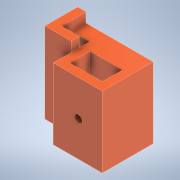
# Autodesk Inventor part: Base Idler Izq
Saved by Autodesk Inventor 2021 (Build 250183000, 183)
## iProperties
Created: 2023-01-27
Part Number: Base Idler Izq
Material: Resina fenólica
Document SubType Name: Modeling
Designer: Diego.labarca
Density: 1.38 g/cm^3
Appearance: Suave - Naranja claro
Author: Diego.labarca
Autodesk Inventor part; units mm, degrees
ref_plane "YZ Plane" through (0, 0, 0) normal (1, 0, 0) x (0, 1, 0)
ref_plane "XZ Plane" through (0, 0, 0) normal (0, 1, 0) x (-1, 0, 0)
ref_plane "XY Plane" through (0, 0, 0) normal (0, 0, 1) x (1, 0, 0)
sketch "Boceto15" plane through (0, 0, 0) normal (1, 0, 0) x (0, 1, 0)
  line L0 (24.65, 10) -> (-24.65, 10)
  line L1 (-24.65, 10) -> (-24.65, -10)
  line L2 (-24.65, -10) -> (24.65, -10)
  line L3 (24.65, -10) -> (24.65, 10)
  line L4 (0, -2.1261) -> (0, 0)
  line L5 (0, 0) -> (1.5481, 0)
  dimension "d52" = 49.3
  dimension "d53" = 20
  constraints: 12 end point, 2 parallel, 2 perpendicular, 1 horizontal, 1 vertical, 2 other
  measures "d52" distance of L2.end L1.end
  measures "d53" distance of L1.end L0.end
extrude "Extrusión12" add sketch "Boceto15" along normal blind 5
sketch "Boceto16" plane through (5, 0, 0) normal (1, 0, 0) x (0, 0, -1)
  circle A0 centre (3.5, -14.65) radius 1.5
  line L0 (10, -24.65) -> (10, 24.65) projected
  line L1 (-10, -24.65) -> (10, -24.65) projected
  circle A1 centre (3.5, 7.35) radius 1.5
  point P0 (0, 0)
  dimension "d56" = 6.5
  dimension "d57" = 10
  dimension "d58" = 3
  dimension "d59" = 3
  dimension "d60" = 32
  dimension "d61" = 6.5
  constraints: 2 centre point
  measures "d56" distance from line of A0.centre L0
  measures "d57" distance from line of L1 A0.centre
  measures "d58" diameter of A0
  measures "d59" diameter of A1
  measures "d60" distance from line of L1 A1.centre
  measures "d61" distance from line of A1.centre L0
extrude "Extrusión13" cut sketch "Boceto16" against normal through all
sketch "Boceto17" plane through (0, -24.65, -10) normal (0, -1, 0) x (1, 0, 0)
  line L0 (5, 20) -> (5, 0) projected
  line L1 (5, 20) -> (16, 20)
  line L2 (16, 20) -> (16, 15)
  line L3 (16, 15) -> (5, 15)
  line L4 (5, 15) -> (5, 20)
  line L5 (16, 15) -> (21, 15)
  line L6 (21, 15) -> (21, 31)
  line L7 (21, 31) -> (16, 31)
  line L8 (16, 31) -> (16, 15)
  line L9 (21, 31) -> (41, 31)
  line L10 (41, 31) -> (41, 26)
  line L11 (41, 26) -> (21, 26)
  line L12 (21, 26) -> (21, 31)
  point P0 (0, 10)
  dimension "d64" = 11
  dimension "d65" = 5
  dimension "d66" = 5
  dimension "d67" = 16
  dimension "d91" = 20
  dimension "d92" = 5
  constraints: 24 end point, 6 parallel, 3 horizontal, 3 perpendicular
  measures "d64" distance of L2.end L3.end
  measures "d65" distance of L1.end L2.end
  measures "d66" distance of L7.end L6.end
  measures "d67" distance of L6.end L5.end
  measures "d91" distance of L10.end L11.end
  measures "d92" distance of L9.end L10.end
extrude "Extrusión14" add sketch "Boceto17" against normal up to surface (49.3 mm away)
sketch "Boceto18" plane through (0, -24.65, 10) normal (0, 0, 1) x (1, 0, 0)
  circle A0 centre (10, 24.3) radius 3.134
  line L0 (0, 0) -> (16, 0) projected
  line L1 (0, 49.3) -> (0, 0) projected
  point P0 (0, 24.65)
  dimension "d70" = 24.3
  dimension "d71" = 10
  constraints: 1 centre point
  measures "d70" distance from line of A0.centre L0
  measures "d71" distance from line of L1 A0.centre
extrude "Extrusión15" cut sketch "Boceto18" against normal up to surface (5 mm away)
sketch "Boceto19" plane through (5, 0, 0) normal (1, 0, 0) x (0, 0, -1)
  line L0 (10, -24.65) -> (10, 24.65) projected
  line L1 (10, -22) -> (7, -22)
  line L2 (7, -22) -> (7, -16)
  line L3 (7, -16) -> (10, -16)
  line L4 (10, -16) -> (10, -22)
  line L5 (10, 9) -> (7, 9)
  line L6 (7, 9) -> (7, 15)
  line L7 (7, 15) -> (10, 15)
  line L8 (10, 15) -> (10, 9)
  line L9 (7, 12) -> (8.4797, 12)
  line L10 (7, -19) -> (9.1788, -19)
  line L11 (-5, -24.65) -> (10, -24.65) projected
  point P0 (0, 0)
  dimension "d74" = 5.65
  dimension "d75" = 6
  dimension "d76" = 6
  dimension "d77" = 31
  dimension "d78" = 3
  constraints: 20 end point, 4 horizontal, 4 parallel, 3 point on line, 2 midpoint, 2 perpendicular
  measures "d74" distance between parallel lines of L11 L10
  measures "d75" distance of L1.end L2.end
  measures "d76" distance of L5.end L6.end
  measures "d77" distance between parallel lines of L10 L9
  measures "d78" distance of L2.end L3.end
extrude "Extrusión16" cut sketch "Boceto19" against normal through all
sketch "Boceto20" plane through (21, -24.65, 5) normal (0, 0, -1) x (-1, 0, 0)
  line L0 (16, 49.3) -> (16, 0) projected
  line L1 (5, 0) -> (5, 49.3) projected
  line L2 (2, 0) -> (2, 49.3)
  line L3 (16, 8.65) -> (16, 33.65) projected
  line L4 (2, 28.65) -> (16, 28.65)
  line L5 (16, 28.65) -> (16, 13.65)
  line L6 (16, 13.65) -> (0, 13.65)
  line L7 (2, 13.65) -> (2, 28.65)
  line L8 (21, 33.65) -> (16, 33.65) projected
  point P0 (2, 13.65)
  dimension "d85" = 5
  dimension "d86" = 15
  dimension "d94" = 14
  constraints: 10 end point, 2 parallel, 2 point on line, 1 horizontal, 1 perpendicular
  measures "d85" distance between parallel lines of L4 L8
  measures "d86" distance between parallel lines of L4 L6
  measures "d94" distance between parallel lines of L0 L7
extrude "Extrusión17" add sketch "Boceto20" along normal up to surface (15 mm away)
sketch "Boceto21" plane through (0, -16, -10) normal (0, 0, -1) x (-1, 0, 0)
  circle A0 centre (-10, 15.65) radius 3.134 projected
  circle A1 centre (-14, 15.65) radius 2
  line L0 (-14, 15.65) -> (-14.5246, 15.65)
  line L1 (-10, 15.65) -> (-9.1195, 15.65)
  line L2 (-21, -8.65) -> (-21, 40.65) projected
  point P0 (0, 16)
  dimension "d87" = 4
  dimension "d106" = 7
  constraints: 4 end point, 2 horizontal, 1 centre point, 1 collinear
  measures "d87" diameter of A1
  measures "d106" distance from line of L2 L0.start
extrude "Extrusión18" cut sketch "Boceto21" against normal blind 7 contours A1 A0 | A0 A1 picked at (-12.7449, 15.65) picked at (-14.0736, 15.5709)
sketch "Boceto22" plane through (0, -24.65, -10) normal (0, -1, 0) x (1, 0, 0)
  line L0 (21, 15) -> (21, 26) projected
  line L1 (21, 13.5) -> (41, 13.5)
  line L2 (41, 13.5) -> (41, 8.5)
  line L3 (41, 8.5) -> (21, 8.5)
  line L4 (21, 8.5) -> (21, 13.5)
  line L5 (21, 26) -> (41, 26) projected
  line L6 (16, 31) -> (16, 20) projected
  line L7 (21, 8.5) -> (16, 8.5)
  line L8 (16, 8.5) -> (16, 20)
  line L9 (16, 20) -> (21, 20)
  line L10 (21, 20) -> (21, 8.5)
  point P0 (0, 10)
  dimension "d95" = 5
  dimension "d96" = 12.5
  constraints: 16 end point, 4 parallel, 2 horizontal, 2 perpendicular, 1 point on line
  measures "d95" distance of L1.end L2.end
  measures "d96" distance between parallel lines of L5 L1
extrude "Extrusión19" add sketch "Boceto22" against normal up to surface (49.3 mm away)
sketch "Boceto24" plane through (41, -24.65, 3.5) normal (1, 0, 0) x (0, 0, -1)
  line L0 (-17.5, 0) -> (-17.5, 49.3) projected
  line L1 (5, 0) -> (5, 49.3) projected
  line L2 (-17.5, 0) -> (5, 0)
  line L3 (5, 0) -> (5, 49.3)
  line L4 (5, 49.3) -> (-17.5, 49.3)
  line L5 (-17.5, 49.3) -> (-17.5, 0)
  point P0 (3.5, 24.65)
  constraints: 8 end point, 2 parallel, 1 horizontal, 1 perpendicular
extrude "Extrusión21" add sketch "Boceto24" along normal blind 5
sketch "Boceto26" plane through (46, -24.65, 3.5) normal (1, 0, 0) x (0, 0, -1)
  line L0 (-17.5, 49.3) -> (-6.5, 49.3) projected
  line L1 (5, 28.65) -> (5, 49.3) projected
  line L2 (-17.5, 49.3) -> (5, 49.3)
  line L3 (5, 49.3) -> (5, 43.3)
  line L4 (5, 43.3) -> (-17.5, 43.3)
  line L5 (-17.5, 43.3) -> (-17.5, 49.3)
  point P0 (3.5, 24.65)
  point P1 (-6.5, 49.3)
  dimension "d111" = 6
  constraints: 8 end point, 2 parallel, 1 horizontal, 1 perpendicular, 1 point on line
  measures "d111" distance of L2.end L3.end
extrude "Extrusión23" cut sketch "Boceto26" against normal up to surface (30 mm away)
sketch "Boceto25" plane through (19, -11, -10) normal (1, 0, 0) x (0, 0, -1)
  line L0 (-15, -13.65) -> (0, -13.65) projected
  line L1 (-8.5, -13.65) -> (-8.5, 0) projected
  line L2 (0, -13.65) -> (-8.5, -13.65)
  line L3 (-8.5, -13.65) -> (-8.5, -6.65)
  line L4 (-8.5, -6.65) -> (0, -6.65)
  line L5 (0, -6.65) -> (0, -13.65)
  line L6 (-8.5, 0) -> (0, 0) projected
  line L7 (0, 0) -> (-3, 0)
  line L8 (-3, 0) -> (-3, -6.65)
  line L9 (-3, -6.65) -> (0, -6.65)
  line L10 (0, -6.65) -> (0, 0)
  line L11 (-8.5, 15) -> (-8.5, 29.65) projected
  line L12 (-8.5, 29.65) -> (0, 29.65)
  line L13 (0, 29.65) -> (0, 22.65)
  line L14 (0, 22.65) -> (-8.5, 22.65)
  line L15 (-8.5, 22.65) -> (-8.5, 29.65)
  line L16 (-8.5, 15) -> (0, 15) projected
  line L17 (0, 22.65) -> (-3, 22.65)
  line L18 (-3, 22.65) -> (-3, 15)
  line L19 (-3, 15) -> (0, 15)
  line L20 (0, 15) -> (0, 22.65)
  point P0 (-10, 11)
  point P1 (0, -6.65)
  point P2 (-3, 0)
  dimension "d107" = 7
  dimension "d108" = 3
  dimension "d114" = 7
  constraints: 32 end point, 8 parallel, 4 horizontal, 4 perpendicular, 3 point on line
  measures "d107" distance of L2.end L3.end
  measures "d108" distance of L9.end L8.end
  measures "d114" distance of L12.end L13.end
extrude "Extrusión22" add sketch "Boceto25" against normal up to surface (14 mm away) contours L1 L4 L5 L0 | L4 L8 L6 L10 | L11 L12 L13 L14 | L18 L14 L20 L16
sketch "Boceto27" plane through (0, -24.65, -10) normal (0, -1, 0) x (1, 0, 0)
  line L0 (19, 0) -> (19, 8.5) projected
  line L1 (46, 8.5) -> (46, 31) projected
  line L2 (19, 0) -> (46, 0)
  line L3 (46, 0) -> (46, 8.5)
  line L4 (46, 8.5) -> (19, 8.5)
  line L5 (19, 8.5) -> (19, 0)
  point P0 (0, 10)
  constraints: 8 end point, 2 parallel, 1 horizontal, 1 perpendicular
extrude "Extrusión24" add sketch "Boceto27" against normal up to surface (43.3 mm away)
sketch "Boceto23" plane through (16, -24.65, 21) normal (0, 0, 1) x (1, 0, 0)
  circle A0 centre (15.15, 21.15) radius 2.5
  line L0 (0, 0) -> (0, 49.3) projected
  line L1 (25, 0) -> (0, 0) projected
  point P0 (-16, 24.65)
  dimension "d99" = 15.15
  dimension "d100" = 21.15
  dimension "d103" = 5
  constraints: 1 centre point
  measures "d99" distance from line of L0 A0.centre
  measures "d100" distance from line of L1 A0.centre
  measures "d103" diameter of A0
extrude "Extrusión20" cut sketch "Boceto23" against normal through all
sketch "Boceto28" plane through (5, 24.65, -10) normal (0, 0, -1) x (-1, 0, 0)
  circle A0 centre (-26.15, -28.15) radius 2.5 projected
  circle A1 centre (-26.15, -28.15) radius 3.5
  point P0 (5, -24.65)
  dimension "d117" = 7
  constraints: 1 centre point, 1 coincident
  measures "d117" diameter of A1
extrude "Extrusión25" cut sketch "Boceto28" against normal blind 7
equation "\"d59\" = d58"
equation "\"d61\" = d56"
equation "\"d76\" = d75"
